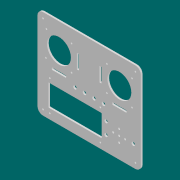
# Autodesk Inventor part: Front
Saved by Autodesk Inventor 2020.1 (Build 241239000, 239)
## iProperties
Created: 2019-07-21
Part Number: Front
Material: Generic
Document SubType Name: Modeling
Designer: Pluscrafter
Density: 1 g/cm^3
Appearance: Default
Author: Pluscrafter
Autodesk Inventor part; units mm, degrees
ref_plane "YZ Plane" through (0, 0, 0) normal (1, 0, 0) x (0, 1, 0)
ref_plane "XZ Plane" through (0, 0, 0) normal (0, 1, 0) x (-1, 0, 0)
ref_plane "XY Plane" through (0, 0, 0) normal (0, 0, 1) x (1, 0, 0)
sketch "Sketch1" plane through (0, 0, 0) normal (0, 0, 1) x (1, 0, 0)
  line L0 (-3, 166.036) -> (167, 166.036)
  line L1 (177, 156.036) -> (177, 11.036)
  line L2 (167, 1.036) -> (-3, 1.036)
  line L3 (-13, 11.036) -> (-13, 156.036)
  arc A0 (177, 156.036) -> (167, 166.036) centre (167, 156.036) ccw
  arc A1 (-3, 166.036) -> (-13, 156.036) centre (-3, 156.036) ccw
  arc A2 (-13, 11.036) -> (-3, 1.036) centre (-3, 11.036) ccw
  arc A3 (167, 1.036) -> (177, 11.036) centre (167, 11.036) ccw
  circle A4 centre (26.45, 119.036) radius 22
  circle A5 centre (137.55, 119.036) radius 22
  line L4 (59.95, 132.136) -> (62.7, 132.136)
  line L5 (63.2, 131.636) -> (63.2, 106.436)
  line L6 (62.7, 105.936) -> (59.95, 105.936)
  line L7 (59.45, 106.436) -> (59.45, 131.636)
  line L8 (101.3, 132.136) -> (104.05, 132.136)
  line L9 (104.55, 131.636) -> (104.55, 106.436)
  line L10 (104.05, 105.936) -> (101.3, 105.936)
  line L11 (100.8, 106.436) -> (100.8, 131.636)
  line L12 (13.85, 86.036) -> (39.05, 86.036)
  line L13 (39.55, 85.536) -> (39.55, 82.786)
  line L14 (39.05, 82.286) -> (13.85, 82.286)
  line L15 (13.35, 82.786) -> (13.35, 85.536)
  line L16 (124.95, 86.036) -> (150.15, 86.036)
  line L17 (150.65, 85.536) -> (150.65, 82.786)
  line L18 (150.15, 82.286) -> (124.95, 82.286)
  line L19 (124.45, 82.786) -> (124.45, 85.536)
  line L20 (26.45, 119.036) -> (137.55, 119.036) construction
  arc A6 (59.95, 132.136) -> (59.45, 131.636) centre (59.95, 131.636) ccw
  arc A7 (63.2, 131.636) -> (62.7, 132.136) centre (62.7, 131.636) ccw
  arc A8 (62.7, 105.936) -> (63.2, 106.436) centre (62.7, 106.436) ccw
  arc A9 (59.45, 106.436) -> (59.95, 105.936) centre (59.95, 106.436) ccw
  arc A10 (100.8, 106.436) -> (101.3, 105.936) centre (101.3, 106.436) ccw
  arc A11 (104.05, 105.936) -> (104.55, 106.436) centre (104.05, 106.436) ccw
  arc A12 (101.3, 132.136) -> (100.8, 131.636) centre (101.3, 131.636) ccw
  arc A13 (104.55, 131.636) -> (104.05, 132.136) centre (104.05, 131.636) ccw
  arc A14 (39.55, 85.536) -> (39.05, 86.036) centre (39.05, 85.536) ccw
  arc A15 (39.05, 82.286) -> (39.55, 82.786) centre (39.05, 82.786) ccw
  arc A16 (13.35, 82.786) -> (13.85, 82.286) centre (13.85, 82.786) ccw
  arc A17 (13.85, 86.036) -> (13.35, 85.536) centre (13.85, 85.536) ccw
  circle A18 centre (49.55, 142.286) radius 1.5
  circle A19 centre (3.35, 142.286) radius 1.5
  circle A20 centre (49.55, 95.786) radius 1.5
  circle A21 centre (2.35, 95.786) radius 1.5
  line L21 (49.55, 142.286) -> (49.55, 95.786) construction
  line L22 (49.55, 142.286) -> (3.35, 142.286) construction
  arc A22 (124.95, 86.036) -> (124.45, 85.536) centre (124.95, 85.536) ccw
  arc A23 (124.45, 82.786) -> (124.95, 82.286) centre (124.95, 82.786) ccw
  arc A24 (150.15, 82.286) -> (150.65, 82.786) centre (150.15, 82.786) ccw
  arc A25 (150.65, 85.536) -> (150.15, 86.036) centre (150.15, 85.536) ccw
  circle A26 centre (114.45, 142.286) radius 1.5
  circle A27 centre (160.65, 142.286) radius 1.5
  circle A28 centre (160.65, 95.786) radius 1.5
  circle A29 centre (114.45, 95.786) radius 1.5
  line L23 (160.65, 142.286) -> (160.65, 95.786) construction
  line L24 (114.45, 142.286) -> (160.65, 142.286) construction
  line L25 (8, 59.036) -> (104, 59.036)
  line L26 (105, 58.036) -> (105, 20.036)
  line L27 (104, 19.036) -> (8, 19.036)
  line L28 (7, 20.036) -> (7, 58.036)
  arc A30 (8, 59.036) -> (7, 58.036) centre (8, 58.036) ccw
  arc A31 (7, 20.036) -> (8, 19.036) centre (8, 20.036) ccw
  arc A32 (104, 19.036) -> (105, 20.036) centre (104, 20.036) ccw
  arc A33 (105, 58.036) -> (104, 59.036) centre (104, 58.036) ccw
  circle A34 centre (55.75, 75.336) radius 3.25
  circle A35 centre (73.25, 75.336) radius 3.25
  circle A36 centre (90.75, 75.336) radius 3.25
  circle A37 centre (108.25, 75.336) radius 3.25
  line L29 (73.25, 75.336) -> (90.75, 75.336) construction
  line L30 (39.55, 82.286) -> (124.45, 82.286) construction
  circle A38 centre (113, 50.036) radius 3.075
  circle A39 centre (113, 28.036) radius 3.075
  line L31 (113, 50.036) -> (113, 28.036) construction
  circle A40 centre (137, 50.036) radius 1.85
  circle A41 centre (126, 39.036) radius 1.85
  circle A42 centre (137, 39.036) radius 1.85
  circle A43 centre (137, 28.036) radius 1.85
  circle A44 centre (148, 39.036) radius 1.85
  circle A45 centre (163, 39.036) radius 3.25
  circle A46 centre (167, 156.036) radius 1.5
  circle A47 centre (-3, 156.036) radius 1.5
  circle A48 centre (167, 11.036) radius 1.5
  circle A49 centre (-3, 11.036) radius 1.5
  circle A50 centre (9.5, 67.036) radius 1.5
  circle A51 centre (102.5, 67.036) radius 1.5
  circle A52 centre (9.5, 11.036) radius 1.5
  circle A53 centre (102.5, 11.036) radius 1.5
  point P0 (0, 0)
  point P1 (-13, 166.036)
  point P2 (177, 1.036)
  point P3 (-13, 1.036)
  point P4 (59.45, 132.136)
  point P5 (63.2, 105.936)
  point P6 (63.2, 132.136)
  point P7 (100.8, 132.136)
  point P8 (104.55, 105.936)
  point P9 (104.55, 132.136)
  point P10 (13.35, 86.036)
  point P11 (13.35, 82.286)
  point P12 (124.45, 86.036)
  point P13 (150.65, 82.286)
  point P14 (104.55, 119.036)
  point P15 (63.2, 119.036)
  point P16 (26.45, 86.036)
  point P17 (137.55, 86.036)
  point P18 (26.45, 142.286)
  point P19 (49.55, 119.036)
  point P20 (160.65, 119.036)
  point P21 (137.55, 142.286)
  point P22 (105, 19.036)
  point P23 (105, 59.036)
  point P24 (7, 19.036)
  point P25 (82, 75.336)
  point P26 (82, 82.286)
  point P27 (113, 39.036)
  point P28 (105, 39.036)
  dimension "d0" = 190
  dimension "d1" = 165
  dimension "d2" = 10
  dimension "d3" = 44
  dimension "d4" = 44
  dimension "d5" = 111.1
  dimension "d6" = 39.45
  dimension "d7" = 39.45
  dimension "d8" = 47
  dimension "d9" = 3.75
  dimension "d10" = 26.2
  dimension "d11" = 3.75
  dimension "d12" = 26.2
  dimension "d13" = 3.75
  dimension "d14" = 26.2
  dimension "d15" = 3.75
  dimension "d16" = 26.2
  dimension "d17" = 33
  dimension "d18" = 33
  dimension "d19" = 33
  dimension "d20" = 33
  dimension "d21" = 0.5
  dimension "a" = 3
  dimension "d23" = 3
  dimension "d24" = 3
  dimension "d25" = 3
  dimension "d26" = 46.2
  dimension "d27" = 47.2
  dimension "d28" = 46.5
  dimension "d29" = 0.5
  dimension "d30" = 3
  dimension "d31" = 3
  dimension "d32" = 3
  dimension "d33" = 3
  dimension "d34" = 46.2
  dimension "d35" = 46.5
  dimension "d36" = 98
  dimension "d37" = 40
  dimension "d38" = 20
  dimension "d39" = 18
  dimension "d40" = 1
  dimension "d41" = 23.25
  dimension "b" = 6.5
  dimension "d43" = 6.5
  dimension "d44" = 6.5
  dimension "d45" = 6.5
  dimension "d" = 17.5
  dimension "d47" = 17.5
  dimension "d48" = 17.5
  dimension "d49" = 16.3
  dimension "e" = 6.15
  dimension "d51" = 6.15
  dimension "d52" = 22
  dimension "d53" = 8
  dimension "i" = 3.7
  dimension "d55" = 3.7
  dimension "d56" = 3.7
  dimension "d57" = 3.7
  dimension "d58" = 3.7
  dimension "d59" = 22
  dimension "d60" = 11
  dimension "d61" = 22
  dimension "d62" = 11
  dimension "d68" = 6.5
  constraints: 64 end point, 54 centre point, 48 point on circle, 48 tangent, 36 point on line, 20 equal radius, 18 horizontal alignment, 12 midpoint, 12 parallel, 11 vertical alignment, 9 horizontal, 7 perpendicular, 4 coincident, 3 vertical
  measures "d0" distance of point (177, 1.036) point (-13, 1.036)
  measures "d1" distance of point (-13, 1.036) point (-13, 166.036)
  measures "d2" radius of A0
  measures "d3" diameter of A4
  measures "d4" diameter of A5
  measures "d5" distance of L20.end L20.start
  measures "d6" distance from line of L3 L20.start
  measures "d7" distance from line of L1 L20.end
  measures "d8" distance from line of L0 L20.start
  measures "d9" distance of point (59.45, 132.136) point (63.2, 132.136)
  measures "d10" distance of point (63.2, 132.136) point (63.2, 105.936)
  measures "d11" distance of point (100.8, 132.136) point (104.55, 132.136)
  measures "d12" distance of point (104.55, 132.136) point (104.55, 105.936)
  measures "d13" distance of point (13.35, 82.286) point (13.35, 86.036)
  measures "d14" distance of L30.start point (13.35, 82.286)
  measures "d15" distance of L30.end point (124.45, 86.036)
  measures "d16" distance of point (150.65, 82.286) L30.end
  measures "d17" distance from line of L12 L20.start
  measures "d18" distance from line of L20.end L16
  measures "d19" distance from line of L20.start L7
  measures "d20" distance from line of L9 L20.end
  measures "d21" radius of A6
  measures "a" diameter of A19
  measures "d23" diameter of A18
  measures "d24" diameter of A21
  measures "d25" diameter of A20
  measures "d26" distance of L21.start L22.end
  measures "d27" distance of L21.end A21.centre
  measures "d28" distance of L21.end L21.start
  measures "d29" radius of A22
  measures "d30" diameter of A26
  measures "d31" diameter of A27
  measures "d32" diameter of A28
  measures "d33" diameter of A29
  measures "d34" distance of L23.start L24.start
  measures "d35" distance of L23.start L23.end
  measures "d36" distance of point (105, 19.036) point (7, 19.036)
  measures "d37" distance of point (105, 59.036) point (105, 19.036)
  measures "d38" distance between parallel lines of L3 L28
  measures "d39" distance between parallel lines of L2 L27
  measures "d40" radius of A30
  measures "d41" distance between parallel lines of L25 L14
  measures "b" diameter of A34
  measures "d43" diameter of A35
  measures "d44" diameter of A36
  measures "d45" diameter of A37
  measures "d" distance of L29.start A34.centre
  measures "d47" distance of L29.end L29.start
  measures "d48" distance of A37.centre L29.end
  measures "d49" distance from line of L25 A34.centre
  measures "e" diameter of A38
  measures "d51" diameter of A39
  measures "d52" distance of L31.end L31.start
  measures "d53" distance from line of L26 point (113, 39.036)
  measures "i" diameter of A40
  measures "d55" diameter of A41
  measures "d56" diameter of A42
  measures "d57" diameter of A43
  measures "d58" diameter of A44
  measures "d59" distance of A43.centre A40.centre
  measures "d60" distance of A43.centre A42.centre
  measures "d61" distance of A41.centre A44.centre
  measures "d62" distance of A41.centre A42.centre
  measures "d68" diameter of A45
extrude "Extrusion1" add sketch "Sketch1" along normal blind 3 contours L0 A0 L1 A3 L2 A2 L3 A1 | A50 | A51 | A52 | A53
extrude "Extrusion2" cut sketch "Sketch1" along normal blind 3 contours A50 | A51 | A52 | A53
equation "\"d23\" = a"
equation "\"d24\" = a"
equation "\"d25\" = a"
equation "\"d30\" = a"
equation "\"d31\" = a"
equation "\"d32\" = a"
equation "\"d33\" = a"
equation "\"d43\" = b"
equation "\"d44\" = b"
equation "\"d45\" = b"
body "Solid1"
